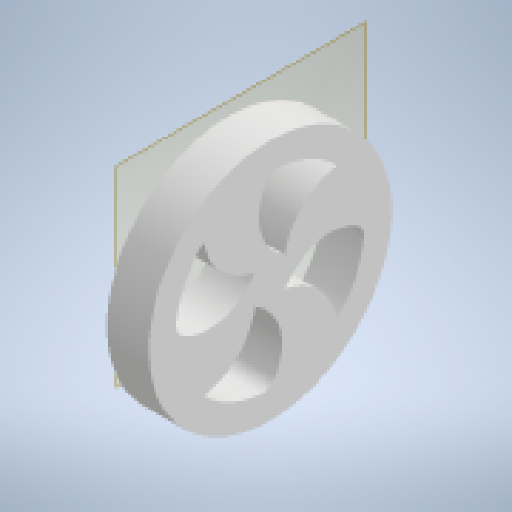
# Autodesk Inventor part: 바퀴
Saved by Autodesk Inventor 2025 (Build 290162010, 162A)
## iProperties
Created: 2024-05-29
Part Number: 바퀴
Material: 일반
Document SubType Name: Modeling
Designer: user
Density: 1 g/cm^3
Appearance: 기본값
Author: user
Autodesk Inventor part; units mm, degrees
ref_plane "YZ Plane" through (0, 0, 0) normal (1, 0, 0) x (0, 1, 0)
ref_plane "XZ Plane" through (0, 0, 0) normal (0, 1, 0) x (-1, 0, 0)
ref_plane "XY Plane" through (0, 0, 0) normal (0, 0, 1) x (1, 0, 0)
ref_plane "작업 평면1" through (-380, -430.4083, 1686.95) normal (1, 0, 0) x (0, 1, 0)
sketch "스케치1" plane through (-380, -430.4083, 1686.95) normal (1, 0, 0) x (0, 1, 0)
  circle A0 centre (0, 0) radius 290
  point P0 (430.4083, -1686.95)
  dimension "d0" = 580
  constraints: 1 centre point
  measures "d0" diameter of A0
extrude "돌출1" add sketch "스케치1" along normal blind 100
sketch "스케치3" plane through (-280, -430.4083, 1686.95) normal (1, 0, 0) x (0, 0, -1)
  circle A0 centre (0, 0) radius 225
  circle A1 centre (0, 0) radius 20 projected
  circle A2 centre (0, 0) radius 50
  arc A3 (225, 0) -> (50, 0) centre (137.5, -121.8349) ccw
  arc A4 (0, -225) -> (0, -50) centre (-121.8349, -137.5) ccw
  line L0 (0, 0) -> (159.099, -159.099)
  line L1 (0, 0) -> (225, 0) construction
  line L2 (159.099, -159.099) -> (-159.099, 159.099)
  line L3 (0, 0) -> (159.099, 159.099)
  line L4 (0, 0) -> (225, 0) construction
  line L5 (159.099, 159.099) -> (-159.099, -159.099)
  arc A5 (-159.099, -159.099) -> (-35.3553, -35.3553) centre (-183.3775, -11.0769) ccw
  arc A6 (159.099, 159.099) -> (35.3553, 35.3553) centre (183.3775, 11.0769) ccw
  arc A7 (159.099, -159.099) -> (35.3553, -35.3553) centre (11.0769, -183.3775) ccw
  arc A8 (-225, 0) -> (-50, 0) centre (-137.5, 121.8349) ccw
  arc A9 (-159.099, 159.099) -> (-35.3553, 35.3553) centre (-11.0769, 183.3775) ccw
  arc A10 (0, 225) -> (0, 50) centre (121.8349, 137.5) ccw
  point P0 (1686.95, 430.4083)
  dimension "d6" = 450
  dimension "d7" = 100
  dimension "d10" = 150
  dimension "d11" = 150
  dimension "d12" = 45
  dimension "d13" = 45
  dimension "d14" = 150
  dimension "d16" = 150
  dimension "d17" = 150
  dimension "d18" = 150
  dimension "d19" = 150
  dimension "d20" = 150
  constraints: 16 point on circle, 12 end point, 8 centre point, 6 point on line, 2 equal length, 2 horizontal, 1 coincident, 20 other
  measures "d10" radius of A3
  measures "d11" radius of A4
  measures "d12" angle of L0 L1
  measures "d13" angle of L4 L3
  measures "d14" radius of A5
  measures "d16" radius of A6
  measures "d17" radius of A7
  measures "d18" radius of A8
  measures "d19" radius of A9
  measures "d20" radius of A10
extrude "돌출3" cut sketch "스케치3" against normal blind 100 contours A0 A7 A2 A3 | A6 A2 A10 A0 | A0 A5 A2 A4 | A9 A2 A8 A0
fillet "모깎기1" radius 121.75 4 edges at (-330, -380.4083, 1686.95) (-330, -430.4083, 1736.95) (-330, -480.4083, 1686.95) (-330, -430.4083, 1636.95)
fillet "모깎기2" radius 36.25 4 edges at (-330, -205.4083, 1686.95) (-330, -430.4083, 1911.95) (-330, -430.4083, 1461.95) (-330, -655.4083, 1686.95)
sketch "스케치4" plane through (-280, -430.4083, 1686.95) normal (1, 0, 0) x (0, 0, -1)
  circle A0 centre (0, 0) radius 20
  point P0 (1686.95, 430.4083)
  dimension "d25" = 40
  constraints: 1 centre point
  measures "d25" diameter of A0
extrude "돌출4" add sketch "스케치4" along normal blind 5
